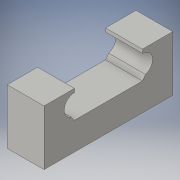
# Autodesk Inventor part: led_clip
Saved by Autodesk Inventor 2016 (Build 200138000, 138)
## iProperties
Created: 2016-02-24
Part Number: led_clip
Material: Generic
Document SubType Name: Modeling
Designer: Matt Ruffner
Density: 1 g/cm^3
Appearance: Default
Author: Matt Ruffner
Autodesk Inventor part; units mm, degrees
ref_plane "YZ Plane" through (0, 0, 0) normal (1, 0, 0) x (0, 1, 0)
ref_plane "XZ Plane" through (0, 0, 0) normal (0, 1, 0) x (-1, 0, 0)
ref_plane "XY Plane" through (0, 0, 0) normal (0, 0, 1) x (1, 0, 0)
sketch "Sketch1" plane through (0, 0, 0) normal (1, 0, 0) x (0, 1, 0)
  line L0 (0, 0) -> (0, -17.78)
  line L1 (0, -17.78) -> (7.62, -17.78)
  line L2 (7.62, -17.78) -> (7.62, -14.986)
  line L3 (0, 0) -> (7.62, 0)
  line L4 (7.62, 0) -> (7.62, -2.794)
  line L5 (3.81, -13.589) -> (3.81, -4.191)
  arc A0 (7.112, -4.191) -> (4.3826, -3.7711) centre (5.715, -4.191) ccw
  arc A1 (4.3826, -14.0089) -> (7.112, -13.589) centre (5.715, -13.589) ccw
  line L6 (7.62, -2.794) -> (7.62, -4.191)
  line L7 (7.62, -4.191) -> (7.112, -4.191)
  line L8 (7.62, -14.986) -> (7.62, -13.589)
  line L9 (7.62, -13.589) -> (7.112, -13.589)
  line L10 (3.81, -4.191) -> (4.3826, -3.7711)
  line L11 (3.81, -13.589) -> (4.3826, -14.0089)
  dimension "d3" = 17.78
  dimension "d4" = 7.62
  dimension "d6" = 2.794
  constraints: 24 end point, 4 point on circle, 4 vertical, 3 horizontal, 2 centre point, 2 perpendicular
  measures "d3" distance of L0.start L0.end
  measures "d4" distance of L0.end L1.end
  measures "d6" distance of L3.end L4.end
extrude "Extrusion1" add sketch "Sketch1" along normal blind 5.08
equation "\"d6\" = d5"
equation "\"d5\" = 2.794"
body "Solid1"
